Autodesk Fusion 360 part; units mm, degrees
(part 4 of 8)
  line L739 (-254.744, -72.9326) -> (-255.545, -72.9326)
  line L740 (-255.545, -72.9326) -> (-255.545, -69.8334)
  line L741 (-255.545, -69.8334) -> (-254.744, -69.8334)
  line L742 (-254.744, -69.8334) -> (-254.744, -64.0334)
  line L743 (-254.744, -64.0334) -> (-255.545, -64.0334)
  line L744 (-255.545, -64.0334) -> (-255.545, -60.9328)
  line L745 (-255.545, -60.9328) -> (-254.744, -60.9328)
  line L746 (-254.744, -60.9328) -> (-254.744, -59.9338)
  line L747 (-254.744, -59.9338) -> (-240.745, -59.9338)
  line L748 (-240.745, -59.9338) -> (-240.745, -60.9328)
  line L749 (-240.745, -60.9328) -> (-239.944, -60.9328)
  line L750 (-239.944, -60.9328) -> (-239.944, -64.0334)
  line L751 (-239.944, -64.0334) -> (-240.745, -64.0334)
  line L752 (-240.745, -64.0334) -> (-240.745, -69.8334)
  line L753 (-240.745, -69.8334) -> (-239.944, -69.8334)
  line L754 (-239.944, -69.8334) -> (-239.944, -72.9326)
  line L755 (-239.944, -72.9326) -> (-240.745, -72.9326)
  line L756 (-252.65, -35.833) -> (-266.65, -35.833)
  line L757 (-266.65, -35.833) -> (-266.65, -31.1326)
  line L758 (-266.65, -31.1326) -> (-268.176, -31.1326)
  line L759 (-268.176, -31.1326) -> (-268.176, -34.3628)
  line L760 (-268.176, -34.3628) -> (-274.925, -34.3628)
  line L761 (-274.925, -34.3628) -> (-274.925, -31.1326)
  line L762 (-274.925, -31.1326) -> (-275.751, -31.1326)
  line L763 (-275.751, -31.1326) -> (-275.751, -28.3338)
  line L764 (-275.751, -28.3338) -> (-274.925, -28.3338)
  line L765 (-274.925, -28.3338) -> (-274.925, -22.0638)
  line L766 (-274.925, -22.0638) -> (-273.2, -22.0638)
  line L767 (-273.2, -22.0638) -> (-273.2, -20.8635)
  line L768 (-273.2, -20.8635) -> (-269.9, -20.8635)
  line L769 (-269.9, -20.8635) -> (-269.9, -22.0638)
  line L770 (-269.9, -22.0638) -> (-268.176, -22.0638)
  line L771 (-268.176, -22.0638) -> (-268.176, -26.5327)
  line L772 (-268.176, -26.5327) -> (-266.65, -26.5327)
  line L773 (-266.65, -26.5327) -> (-266.65, -21.8336)
  line L774 (-266.65, -21.8336) -> (-252.65, -21.8336)
  line L775 (-252.65, -21.8336) -> (-252.65, -26.5327)
  line L776 (-252.65, -26.5327) -> (-251.126, -26.5327)
  line L777 (-251.126, -26.5327) -> (-251.126, -22.0638)
  line L778 (-251.126, -22.0638) -> (-249.4, -22.0638)
  line L779 (-249.4, -22.0638) -> (-249.4, -20.8635)
  line L780 (-249.4, -20.8635) -> (-246.101, -20.8635)
  line L781 (-246.101, -20.8635) -> (-246.101, -22.0638)
  line L782 (-246.101, -22.0638) -> (-244.376, -22.0638)
  line L783 (-244.376, -22.0638) -> (-244.376, -28.3338)
  line L784 (-244.376, -28.3338) -> (-243.55, -28.3338)
  line L785 (-243.55, -28.3338) -> (-243.55, -31.1326)
  line L786 (-243.55, -31.1326) -> (-244.376, -31.1326)
  line L787 (-244.376, -31.1326) -> (-244.376, -34.3628)
  line L788 (-244.376, -34.3628) -> (-251.126, -34.3628)
  line L789 (-251.126, -34.3628) -> (-251.126, -31.1326)
  line L790 (-251.126, -31.1326) -> (-252.65, -31.1326)
  line L791 (-252.65, -31.1326) -> (-252.65, -35.833)
  line L792 (-174.07, -91.9826) -> (-174.07, -92.9831)
  line L793 (-174.07, -92.9831) -> (-188.069, -92.9831)
  line L794 (-188.069, -92.9831) -> (-188.069, -91.9826)
  line L795 (-188.069, -91.9826) -> (-188.87, -91.9826)
  line L796 (-188.87, -91.9826) -> (-188.87, -88.8834)
  line L797 (-188.87, -88.8834) -> (-188.069, -88.8834)
  line L798 (-188.069, -88.8834) -> (-188.069, -83.0834)
  line L799 (-188.069, -83.0834) -> (-188.87, -83.0834)
  line L800 (-188.87, -83.0834) -> (-188.87, -79.9828)
  line L801 (-188.87, -79.9828) -> (-188.069, -79.9828)
  line L802 (-188.069, -79.9828) -> (-188.069, -78.9838)
  line L803 (-188.069, -78.9838) -> (-174.07, -78.9838)
  line L804 (-174.07, -78.9838) -> (-174.07, -79.9828)
  line L805 (-174.07, -79.9828) -> (-173.269, -79.9828)
  line L806 (-173.269, -79.9828) -> (-173.269, -83.0834)
  line L807 (-173.269, -83.0834) -> (-174.07, -83.0834)
  line L808 (-174.07, -83.0834) -> (-174.07, -88.8834)
  line L809 (-174.07, -88.8834) -> (-173.269, -88.8834)
  line L810 (-173.269, -88.8834) -> (-173.269, -91.9826)
  line L811 (-173.269, -91.9826) -> (-174.07, -91.9826)
  line L812 (-188.357, -53.8826) -> (-188.357, -54.8831)
  line L813 (-188.357, -54.8831) -> (-202.357, -54.8831)
  line L814 (-202.357, -54.8831) -> (-202.357, -53.8826)
  line L815 (-202.357, -53.8826) -> (-203.156, -53.8826)
  line L816 (-203.156, -53.8826) -> (-203.156, -50.7834)
  line L817 (-203.156, -50.7834) -> (-202.357, -50.7834)
  line L818 (-202.357, -50.7834) -> (-202.357, -44.9834)
  line L819 (-202.357, -44.9834) -> (-203.156, -44.9834)
  line L820 (-203.156, -44.9834) -> (-203.156, -41.8828)
  line L821 (-203.156, -41.8828) -> (-202.357, -41.8828)
  line L822 (-202.357, -41.8828) -> (-202.357, -40.8838)
  line L823 (-202.357, -40.8838) -> (-188.357, -40.8838)
  line L824 (-188.357, -40.8838) -> (-188.357, -41.8828)
  line L825 (-188.357, -41.8828) -> (-187.556, -41.8828)
  line L826 (-187.556, -41.8828) -> (-187.556, -44.9834)
  line L827 (-187.556, -44.9834) -> (-188.357, -44.9834)
  line L828 (-188.357, -44.9834) -> (-188.357, -50.7834)
  line L829 (-188.357, -50.7834) -> (-187.556, -50.7834)
  line L830 (-187.556, -50.7834) -> (-187.556, -53.8826)
  line L831 (-187.556, -53.8826) -> (-188.357, -53.8826)
  line L832 (-195.501, -15.7827) -> (-195.501, -16.7831)
  line L833 (-195.501, -16.7831) -> (-209.5, -16.7831)
  line L834 (-209.5, -16.7831) -> (-209.5, -15.7827)
  line L835 (-209.5, -15.7827) -> (-210.301, -15.7827)
  line L836 (-210.301, -15.7827) -> (-210.301, -12.6848)
  line L837 (-210.301, -12.6848) -> (-209.5, -12.6848)
  line L838 (-209.5, -12.6848) -> (-209.5, -6.8833)
  line L839 (-209.5, -6.8833) -> (-210.301, -6.8833)
  line L840 (-210.301, -6.8833) -> (-210.301, -3.7827)
  line L841 (-210.301, -3.7827) -> (-209.5, -3.7827)
  line L842 (-209.5, -3.7827) -> (-209.5, -2.7836)
  line L843 (-209.5, -2.7836) -> (-195.501, -2.7836)
  line L844 (-195.501, -2.7836) -> (-195.501, -3.7827)
  line L845 (-195.501, -3.7827) -> (-194.7, -3.7827)
  line L846 (-194.7, -3.7827) -> (-194.7, -6.8833)
  line L847 (-194.7, -6.8833) -> (-195.501, -6.8833)
  line L848 (-195.501, -6.8833) -> (-195.501, -12.6848)
  line L849 (-195.501, -12.6848) -> (-194.7, -12.6848)
  line L850 (-194.7, -12.6848) -> (-194.7, -15.7827)
  line L851 (-194.7, -15.7827) -> (-195.501, -15.7827)
  line L852 (-155.02, -91.9826) -> (-155.02, -92.9831)
  line L853 (-155.02, -92.9831) -> (-169.019, -92.9831)
  line L854 (-169.019, -92.9831) -> (-169.019, -91.9826)
  line L855 (-169.019, -91.9826) -> (-169.82, -91.9826)
  line L856 (-169.82, -91.9826) -> (-169.82, -88.8834)
  line L857 (-169.82, -88.8834) -> (-169.019, -88.8834)
  line L858 (-169.019, -88.8834) -> (-169.019, -83.0834)
  line L859 (-169.019, -83.0834) -> (-169.82, -83.0834)
  line L860 (-169.82, -83.0834) -> (-169.82, -79.9828)
  line L861 (-169.82, -79.9828) -> (-169.019, -79.9828)
  line L862 (-169.019, -79.9828) -> (-169.019, -78.9838)
  line L863 (-169.019, -78.9838) -> (-155.02, -78.9838)
  line L864 (-155.02, -78.9838) -> (-155.02, -79.9828)
  line L865 (-155.02, -79.9828) -> (-154.219, -79.9828)
  line L866 (-154.219, -79.9828) -> (-154.219, -83.0834)
  line L867 (-154.219, -83.0834) -> (-155.02, -83.0834)
  line L868 (-155.02, -83.0834) -> (-155.02, -88.8834)
  line L869 (-155.02, -88.8834) -> (-154.219, -88.8834)
  line L870 (-154.219, -88.8834) -> (-154.219, -91.9826)
  line L871 (-154.219, -91.9826) -> (-155.02, -91.9826)
  line L872 (-159.782, -34.8327) -> (-159.782, -35.833)
  line L873 (-159.782, -35.833) -> (-173.782, -35.833)
  line L874 (-173.782, -35.833) -> (-173.782, -34.8327)
  line L875 (-173.782, -34.8327) -> (-174.581, -34.8327)
  line L876 (-174.581, -34.8327) -> (-174.581, -31.7348)
  line L877 (-174.581, -31.7348) -> (-173.782, -31.7348)
  line L878 (-173.782, -31.7348) -> (-173.782, -25.9333)
  line L879 (-173.782, -25.9333) -> (-174.581, -25.9333)
  line L880 (-174.581, -25.9333) -> (-174.581, -22.8327)
  line L881 (-174.581, -22.8327) -> (-173.782, -22.8327)
  line L882 (-173.782, -22.8327) -> (-173.782, -21.8336)
  line L883 (-173.782, -21.8336) -> (-159.782, -21.8336)
  line L884 (-159.782, -21.8336) -> (-159.782, -22.8327)
  line L885 (-159.782, -22.8327) -> (-158.981, -22.8327)
  line L886 (-158.981, -22.8327) -> (-158.981, -25.9333)
  line L887 (-158.981, -25.9333) -> (-159.782, -25.9333)
  line L888 (-159.782, -25.9333) -> (-159.782, -31.7348)
  line L889 (-159.782, -31.7348) -> (-158.981, -31.7348)
  line L890 (-158.981, -31.7348) -> (-158.981, -34.8327)
  line L891 (-158.981, -34.8327) -> (-159.782, -34.8327)
  line L892 (-116.918, -91.9826) -> (-116.918, -92.9831)
  line L893 (-116.918, -92.9831) -> (-130.919, -92.9831)
  line L894 (-130.919, -92.9831) -> (-130.919, -91.9826)
  line L895 (-130.919, -91.9826) -> (-131.72, -91.9826)
  line L896 (-131.72, -91.9826) -> (-131.72, -88.8834)
  line L897 (-131.72, -88.8834) -> (-130.919, -88.8834)
  line L898 (-130.919, -88.8834) -> (-130.919, -83.0834)
  line L899 (-130.919, -83.0834) -> (-131.72, -83.0834)
  line L900 (-131.72, -83.0834) -> (-131.72, -79.9828)
  line L901 (-131.72, -79.9828) -> (-130.919, -79.9828)
  line L902 (-130.919, -79.9828) -> (-130.919, -78.9838)
  line L903 (-130.919, -78.9838) -> (-116.918, -78.9838)
  line L904 (-116.918, -78.9838) -> (-116.918, -79.9828)
  line L905 (-116.918, -79.9828) -> (-116.119, -79.9828)
  line L906 (-116.119, -79.9828) -> (-116.119, -83.0834)
  line L907 (-116.119, -83.0834) -> (-116.918, -83.0834)
  line L908 (-116.918, -83.0834) -> (-116.918, -88.8834)
  line L909 (-116.918, -88.8834) -> (-116.119, -88.8834)
  line L910 (-116.119, -88.8834) -> (-116.119, -91.9826)
  line L911 (-116.119, -91.9826) -> (-116.918, -91.9826)
  line L912 (-121.682, -34.8327) -> (-121.682, -35.833)
  line L913 (-121.682, -35.833) -> (-135.682, -35.833)
  line L914 (-135.682, -35.833) -> (-135.682, -34.8327)
  line L915 (-135.682, -34.8327) -> (-136.481, -34.8327)
  line L916 (-136.481, -34.8327) -> (-136.481, -31.7348)
  line L917 (-136.481, -31.7348) -> (-135.682, -31.7348)
  line L918 (-135.682, -31.7348) -> (-135.682, -25.9333)
  line L919 (-135.682, -25.9333) -> (-136.481, -25.9333)
  line L920 (-136.481, -25.9333) -> (-136.481, -22.8327)
  line L921 (-136.481, -22.8327) -> (-135.682, -22.8327)
  line L922 (-135.682, -22.8327) -> (-135.682, -21.8336)
  line L923 (-135.682, -21.8336) -> (-121.682, -21.8336)
  line L924 (-121.682, -21.8336) -> (-121.682, -22.8327)
  line L925 (-121.682, -22.8327) -> (-120.881, -22.8327)
  line L926 (-120.881, -22.8327) -> (-120.881, -25.9333)
  line L927 (-120.881, -25.9333) -> (-121.682, -25.9333)
  line L928 (-121.682, -25.9333) -> (-121.682, -31.7348)
  line L929 (-121.682, -31.7348) -> (-120.881, -31.7348)
  line L930 (-120.881, -31.7348) -> (-120.881, -34.8327)
  line L931 (-120.881, -34.8327) -> (-121.682, -34.8327)
  line L932 (-78.8197, -91.9826) -> (-78.8197, -92.9831)
  line L933 (-78.8197, -92.9831) -> (-92.819, -92.9831)
  line L934 (-92.819, -92.9831) -> (-92.819, -91.9826)
  line L935 (-92.819, -91.9826) -> (-93.6184, -91.9826)
  line L936 (-93.6184, -91.9826) -> (-93.6184, -88.8834)
  line L937 (-93.6184, -88.8834) -> (-92.819, -88.8834)
  line L938 (-92.819, -88.8834) -> (-92.819, -83.0834)
  line L939 (-92.819, -83.0834) -> (-93.6184, -83.0834)
  line L940 (-93.6184, -83.0834) -> (-93.6184, -79.9828)
  line L941 (-93.6184, -79.9828) -> (-92.819, -79.9828)
  line L942 (-92.819, -79.9828) -> (-92.819, -78.9838)
  line L943 (-92.819, -78.9838) -> (-78.8197, -78.9838)
  line L944 (-78.8197, -78.9838) -> (-78.8197, -79.9828)
  line L945 (-78.8197, -79.9828) -> (-78.0189, -79.9828)
  line L946 (-78.0189, -79.9828) -> (-78.0189, -83.0834)
  line L947 (-78.0189, -83.0834) -> (-78.8197, -83.0834)
  line L948 (-78.8197, -83.0834) -> (-78.8197, -88.8834)
  line L949 (-78.8197, -88.8834) -> (-78.0189, -88.8834)
  line L950 (-78.0189, -88.8834) -> (-78.0189, -91.9826)
  line L951 (-78.0189, -91.9826) -> (-78.8197, -91.9826)
  line L952 (-83.5822, -34.8327) -> (-83.5822, -35.833)
  line L953 (-83.5822, -35.833) -> (-97.5815, -35.833)
  line L954 (-97.5815, -35.833) -> (-97.5815, -34.8327)
  line L955 (-97.5815, -34.8327) -> (-98.3809, -34.8327)
  line L956 (-98.3809, -34.8327) -> (-98.3809, -31.7348)
  line L957 (-98.3809, -31.7348) -> (-97.5815, -31.7348)
  line L958 (-97.5815, -31.7348) -> (-97.5815, -25.9333)
  line L959 (-97.5815, -25.9333) -> (-98.3809, -25.9333)
  line L960 (-98.3809, -25.9333) -> (-98.3809, -22.8327)
  line L961 (-98.3809, -22.8327) -> (-97.5815, -22.8327)
  line L962 (-97.5815, -22.8327) -> (-97.5815, -21.8336)
  line L963 (-97.5815, -21.8336) -> (-83.5822, -21.8336)
  line L964 (-83.5822, -21.8336) -> (-83.5822, -22.8327)
  line L965 (-83.5822, -22.8327) -> (-82.7814, -22.8327)
  line L966 (-82.7814, -22.8327) -> (-82.7814, -25.9333)
  line L967 (-82.7814, -25.9333) -> (-83.5822, -25.9333)
  line L968 (-83.5822, -25.9333) -> (-83.5822, -31.7348)
  line L969 (-83.5822, -31.7348) -> (-82.7814, -31.7348)
  line L970 (-82.7814, -31.7348) -> (-82.7814, -34.8327)
  line L971 (-82.7814, -34.8327) -> (-83.5822, -34.8327)
  line L972 (-50.2447, -72.9326) -> (-50.2447, -73.9331)
  line L973 (-50.2447, -73.9331) -> (-64.244, -73.9331)
  line L974 (-64.244, -73.9331) -> (-64.244, -72.9326)
  line L975 (-64.244, -72.9326) -> (-65.0448, -72.9326)
  line L976 (-65.0448, -72.9326) -> (-65.0448, -69.8334)
  line L977 (-65.0448, -69.8334) -> (-64.244, -69.8334)
  line L978 (-64.244, -69.8334) -> (-64.244, -64.0334)
  line L979 (-64.244, -64.0334) -> (-65.0448, -64.0334)
  line L980 (-65.0448, -64.0334) -> (-65.0448, -60.9328)
  line L981 (-65.0448, -60.9328) -> (-64.244, -60.9328)
  line L982 (-64.244, -60.9328) -> (-64.244, -59.9338)
  line L983 (-64.244, -59.9338) -> (-50.2447, -59.9338)
  line L984 (-50.2447, -59.9338) -> (-50.2447, -60.9328)
  line L985 (-50.2447, -60.9328) -> (-49.4439, -60.9328)
  line L986 (-49.4439, -60.9328) -> (-49.4439, -64.0334)
  line L987 (-49.4439, -64.0334) -> (-50.2447, -64.0334)
  line L988 (-50.2447, -64.0334) -> (-50.2447, -69.8334)
  line L989 (-50.2447, -69.8334) -> (-49.4439, -69.8334)
  line L990 (-49.4439, -69.8334) -> (-49.4439, -72.9326)
  line L991 (-49.4439, -72.9326) -> (-50.2447, -72.9326)
  line L992 (-45.4822, -34.8327) -> (-45.4822, -35.833)
  line L993 (-45.4822, -35.833) -> (-59.4815, -35.833)
  line L994 (-59.4815, -35.833) -> (-59.4815, -34.8327)
  line L995 (-59.4815, -34.8327) -> (-60.2809, -34.8327)
  line L996 (-60.2809, -34.8327) -> (-60.2809, -31.7348)
  line L997 (-60.2809, -31.7348) -> (-59.4815, -31.7348)
  line L998 (-59.4815, -31.7348) -> (-59.4815, -25.9333)
  line L999 (-59.4815, -25.9333) -> (-60.2809, -25.9333)
  line L1000 (-60.2809, -25.9333) -> (-60.2809, -22.8327)
  line L1001 (-60.2809, -22.8327) -> (-59.4815, -22.8327)
  line L1002 (-59.4815, -22.8327) -> (-59.4815, -21.8336)
  line L1003 (-59.4815, -21.8336) -> (-45.4822, -21.8336)
  line L1004 (-45.4822, -21.8336) -> (-45.4822, -22.8327)
  line L1005 (-45.4822, -22.8327) -> (-44.6814, -22.8327)
  line L1006 (-44.6814, -22.8327) -> (-44.6814, -25.9333)
  line L1007 (-44.6814, -25.9333) -> (-45.4822, -25.9333)
  line L1008 (-45.4822, -25.9333) -> (-45.4822, -31.7348)
  line L1009 (-45.4822, -31.7348) -> (-44.6814, -31.7348)
  line L1010 (-44.6814, -31.7348) -> (-44.6814, -34.8327)
  line L1011 (-44.6814, -34.8327) -> (-45.4822, -34.8327)
  line L1012 (-14.5259, -35.833) -> (-28.5254, -35.833)
  line L1013 (-28.5254, -35.833) -> (-28.5254, -31.1326)
  line L1014 (-28.5254, -31.1326) -> (-30.0509, -31.1326)
  line L1015 (-30.0509, -31.1326) -> (-30.0509, -34.3628)
  line L1016 (-30.0509, -34.3628) -> (-36.8004, -34.3628)
  line L1017 (-36.8004, -34.3628) -> (-36.8004, -31.1326)
  line L1018 (-36.8004, -31.1326) -> (-37.6259, -31.1326)
  line L1019 (-37.6259, -31.1326) -> (-37.6259, -28.3338)
  line L1020 (-37.6259, -28.3338) -> (-36.8004, -28.3338)
  line L1021 (-36.8004, -28.3338) -> (-36.8004, -22.0638)
  line L1022 (-36.8004, -22.0638) -> (-35.0752, -22.0638)
  line L1023 (-35.0752, -22.0638) -> (-35.0752, -20.8635)
  line L1024 (-35.0752, -20.8635) -> (-31.7748, -20.8635)
  line L1025 (-31.7748, -20.8635) -> (-31.7748, -22.0638)
  line L1026 (-31.7748, -22.0638) -> (-30.0509, -22.0638)
  line L1027 (-30.0509, -22.0638) -> (-30.0509, -26.5327)
  line L1028 (-30.0509, -26.5327) -> (-28.5254, -26.5327)
  line L1029 (-28.5254, -26.5327) -> (-28.5254, -21.8336)
  line L1030 (-28.5254, -21.8336) -> (-14.5259, -21.8336)
  line L1031 (-14.5259, -21.8336) -> (-14.5259, -26.5327)
  line L1032 (-14.5259, -26.5327) -> (-13.0004, -26.5327)
  line L1033 (-13.0004, -26.5327) -> (-13.0004, -22.0638)
  line L1034 (-13.0004, -22.0638) -> (-11.2751, -22.0638)
  line L1035 (-11.2751, -22.0638) -> (-11.2751, -20.8635)
  line L1036 (-11.2751, -20.8635) -> (-7.9761, -20.8635)
  line L1037 (-7.9761, -20.8635) -> (-7.9761, -22.0638)
  line L1038 (-7.9761, -22.0638) -> (-6.2508, -22.0638)
  line L1039 (-6.2508, -22.0638) -> (-6.2508, -28.3338)
  line L1040 (-6.2508, -28.3338) -> (-5.4253, -28.3338)
  line L1041 (-5.4253, -28.3338) -> (-5.4253, -31.1326)
  line L1042 (-5.4253, -31.1326) -> (-6.2508, -31.1326)
  line L1043 (-6.2508, -31.1326) -> (-6.2508, -34.3628)
  line L1044 (-6.2508, -34.3628) -> (-13.0004, -34.3628)
  line L1045 (-13.0004, -34.3628) -> (-13.0004, -31.1326)
  line L1046 (-13.0004, -31.1326) -> (-14.5259, -31.1326)
  line L1047 (-14.5259, -31.1326) -> (-14.5259, -35.833)
  line L1048 (-7.3822, -72.9326) -> (-7.3822, -73.9331)
  line L1049 (-7.3822, -73.9331) -> (-21.3817, -73.9331)
  line L1050 (-21.3817, -73.9331) -> (-21.3817, -72.9326)
  line L1051 (-21.3817, -72.9326) -> (-22.1809, -72.9326)
  line L1052 (-22.1809, -72.9326) -> (-22.1809, -69.8334)
  line L1053 (-22.1809, -69.8334) -> (-21.3817, -69.8334)
  line L1054 (-21.3817, -69.8334) -> (-21.3817, -64.0334)
  line L1055 (-21.3817, -64.0334) -> (-22.1809, -64.0334)
  line L1056 (-22.1809, -64.0334) -> (-22.1809, -60.9328)
  line L1057 (-22.1809, -60.9328) -> (-21.3817, -60.9328)
  line L1058 (-21.3817, -60.9328) -> (-21.3817, -59.9338)
  line L1059 (-21.3817, -59.9338) -> (-7.3822, -59.9338)
  line L1060 (-7.3822, -59.9338) -> (-7.3822, -60.9328)
  line L1061 (-7.3822, -60.9328) -> (-6.5815, -60.9328)
  line L1062 (-6.5815, -60.9328) -> (-6.5815, -64.0334)
  line L1063 (-6.5815, -64.0334) -> (-7.3822, -64.0334)
  line L1064 (-7.3822, -64.0334) -> (-7.3822, -69.8334)
  line L1065 (-7.3822, -69.8334) -> (-6.5815, -69.8334)
  line L1066 (-6.5815, -69.8334) -> (-6.5815, -72.9326)
  line L1067 (-6.5815, -72.9326) -> (-7.3822, -72.9326)
  line L1068 (-9.762, -53.8826) -> (-9.762, -54.8831)
  line L1069 (-9.762, -54.8831) -> (-23.7629, -54.8831)
  line L1070 (-23.7629, -54.8831) -> (-23.7629, -53.8826)
  line L1071 (-23.7629, -53.8826) -> (-24.5622, -53.8826)
  line L1072 (-24.5622, -53.8826) -> (-24.5622, -50.7834)
  line L1073 (-24.5622, -50.7834) -> (-23.7629, -50.7834)
  line L1074 (-23.7629, -50.7834) -> (-23.7629, -44.9834)
  line L1075 (-23.7629, -44.9834) -> (-24.5622, -44.9834)
  line L1076 (-24.5622, -44.9834) -> (-24.5622, -41.8828)
  line L1077 (-24.5622, -41.8828) -> (-23.7629, -41.8828)
  line L1078 (-23.7629, -41.8828) -> (-23.7629, -40.8838)
  line L1079 (-23.7629, -40.8838) -> (-9.762, -40.8838)
  line L1080 (-9.762, -40.8838) -> (-9.762, -41.8828)
  line L1081 (-9.762, -41.8828) -> (-8.9628, -41.8828)
  line L1082 (-8.9628, -41.8828) -> (-8.9628, -44.9834)
  line L1083 (-8.9628, -44.9834) -> (-9.762, -44.9834)
  line L1084 (-9.762, -44.9834) -> (-9.762, -50.7834)
  line L1085 (-9.762, -50.7834) -> (-8.9628, -50.7834)
  line L1086 (-8.9628, -50.7834) -> (-8.9628, -53.8826)
  line L1087 (-8.9628, -53.8826) -> (-9.762, -53.8826)
  line L1088 (-52.626, -15.7827) -> (-52.626, -16.7831)
  line L1089 (-52.626, -16.7831) -> (-66.6253, -16.7831)
  line L1090 (-66.6253, -16.7831) -> (-66.6253, -15.7827)
  line L1091 (-66.6253, -15.7827) -> (-67.4261, -15.7827)
  line L1092 (-67.4261, -15.7827) -> (-67.4261, -12.6848)
  line L1093 (-67.4261, -12.6848) -> (-66.6253, -12.6848)
  line L1094 (-66.6253, -12.6848) -> (-66.6253, -6.8833)
  line L1095 (-66.6253, -6.8833) -> (-67.4261, -6.8833)
  line L1096 (-67.4261, -6.8833) -> (-67.4261, -3.7827)
  line L1097 (-67.4261, -3.7827) -> (-66.6253, -3.7827)
  line L1098 (-66.6253, -3.7827) -> (-66.6253, -2.7836)
  line L1099 (-66.6253, -2.7836) -> (-52.626, -2.7836)
  line L1100 (-52.626, -2.7836) -> (-52.626, -3.7827)
  line L1101 (-52.626, -3.7827) -> (-51.8252, -3.7827)
  line L1102 (-51.8252, -3.7827) -> (-51.8252, -6.8833)
  line L1103 (-51.8252, -6.8833) -> (-52.626, -6.8833)
  line L1104 (-52.626, -6.8833) -> (-52.626, -12.6848)
  line L1105 (-52.626, -12.6848) -> (-51.8252, -12.6848)
  line L1106 (-51.8252, -12.6848) -> (-51.8252, -15.7827)
  line L1107 (-51.8252, -15.7827) -> (-52.626, -15.7827)
  line L1108 (-40.7197, -91.9826) -> (-40.7197, -92.9831)
  line L1109 (-40.7197, -92.9831) -> (-54.719, -92.9831)
  line L1110 (-54.719, -92.9831) -> (-54.719, -91.9826)
  line L1111 (-54.719, -91.9826) -> (-55.5198, -91.9826)
  line L1112 (-55.5198, -91.9826) -> (-55.5198, -88.8834)
  line L1113 (-55.5198, -88.8834) -> (-54.719, -88.8834)
  line L1114 (-54.719, -88.8834) -> (-54.719, -83.0834)
  line L1115 (-54.719, -83.0834) -> (-55.5198, -83.0834)
  line L1116 (-55.5198, -83.0834) -> (-55.5198, -79.9828)
  line L1117 (-55.5198, -79.9828) -> (-54.719, -79.9828)
  line L1118 (-54.719, -79.9828) -> (-54.719, -78.9838)
  line L1119 (-54.719, -78.9838) -> (-40.7197, -78.9838)
  line L1120 (-40.7197, -78.9838) -> (-40.7197, -79.9828)
  line L1121 (-40.7197, -79.9828) -> (-39.9189, -79.9828)
  line L1122 (-39.9189, -79.9828) -> (-39.9189, -83.0834)
  line L1123 (-39.9189, -83.0834) -> (-40.7197, -83.0834)
  line L1124 (-40.7197, -83.0834) -> (-40.7197, -88.8834)
  line L1125 (-40.7197, -88.8834) -> (-39.9189, -88.8834)
  line L1126 (-39.9189, -88.8834) -> (-39.9189, -91.9826)
  line L1127 (-39.9189, -91.9826) -> (-40.7197, -91.9826)
  line L1128 (-124.062, -15.7827) -> (-124.062, -16.7831)
  line L1129 (-124.062, -16.7831) -> (-138.063, -16.7831)
  line L1130 (-138.063, -16.7831) -> (-138.063, -15.7827)
  line L1131 (-138.063, -15.7827) -> (-138.862, -15.7827)
  line L1132 (-138.862, -15.7827) -> (-138.862, -12.6848)
  line L1133 (-138.862, -12.6848) -> (-138.063, -12.6848)
  line L1134 (-138.063, -12.6848) -> (-138.063, -12.0826)
  line L1135 (-138.063, -12.0826) -> (-177.687, -12.0826)
  line L1136 (-177.687, -12.0826) -> (-177.687, -15.3128)
  line L1137 (-177.687, -15.3128) -> (-184.438, -15.3128)
  line L1138 (-184.438, -15.3128) -> (-184.438, -12.0826)
  line L1139 (-184.438, -12.0826) -> (-185.262, -12.0826)
  line L1140 (-185.262, -12.0826) -> (-185.262, -9.2838)
  line L1141 (-185.262, -9.2838) -> (-184.438, -9.2838)
  line L1142 (-184.438, -9.2838) -> (-184.438, -3.0138)
  line L1143 (-184.438, -3.0138) -> (-182.713, -3.0138)
  line L1144 (-182.713, -3.0138) -> (-182.713, -1.8135)
  line L1145 (-182.713, -1.8135) -> (-179.412, -1.8135)
  line L1146 (-179.412, -1.8135) -> (-179.412, -3.0138)
  line L1147 (-179.412, -3.0138) -> (-177.687, -3.0138)
  line L1148 (-177.687, -3.0138) -> (-177.687, -7.4841)
  line L1149 (-177.687, -7.4841) -> (-138.063, -7.4841)
  line L1150 (-138.063, -7.4841) -> (-138.063, -6.8833)
  line L1151 (-138.063, -6.8833) -> (-138.862, -6.8833)
  line L1152 (-138.862, -6.8833) -> (-138.862, -3.7827)
  line L1153 (-138.862, -3.7827) -> (-138.063, -3.7827)
  line L1154 (-138.063, -3.7827) -> (-138.063, -2.7836)
  line L1155 (-138.063, -2.7836) -> (-124.062, -2.7836)
  line L1156 (-124.062, -2.7836) -> (-124.062, -3.7827)
  line L1157 (-124.062, -3.7827) -> (-123.263, -3.7827)
  line L1158 (-123.263, -3.7827) -> (-123.263, -6.8833)
  line L1159 (-123.263, -6.8833) -> (-124.062, -6.8833)
  line L1160 (-124.062, -6.8833) -> (-124.062, -7.4841)
  line L1161 (-124.062, -7.4841) -> (-84.4381, -7.4841)
  line L1162 (-84.4381, -7.4841) -> (-84.4381, -3.0138)
  line L1163 (-84.4381, -3.0138) -> (-82.7126, -3.0138)
  line L1164 (-82.7126, -3.0138) -> (-82.7126, -1.8135)
  line L1165 (-82.7126, -1.8135) -> (-79.412, -1.8135)
  line L1166 (-79.412, -1.8135) -> (-79.412, -3.0138)
  line L1167 (-79.412, -3.0138) -> (-77.687, -3.0138)
  line L1168 (-77.687, -3.0138) -> (-77.687, -9.2838)
  line L1169 (-77.687, -9.2838) -> (-76.8629, -9.2838)
  line L1170 (-76.8629, -9.2838) -> (-76.8629, -12.0826)
  line L1171 (-76.8629, -12.0826) -> (-77.687, -12.0826)
  line L1172 (-77.687, -12.0826) -> (-77.687, -15.3128)
  line L1173 (-77.687, -15.3128) -> (-84.4381, -15.3128)
  line L1174 (-84.4381, -15.3128) -> (-84.4381, -12.0826)
  line L1175 (-84.4381, -12.0826) -> (-124.062, -12.0826)
  line L1176 (-124.062, -12.0826) -> (-124.062, -12.6848)
  line L1177 (-124.062, -12.6848) -> (-123.263, -12.6848)
  line L1178 (-123.263, -12.6848) -> (-123.263, -15.7827)
  line L1179 (-123.263, -15.7827) -> (-124.062, -15.7827)
  line L1180 (-59.7697, -91.9826) -> (-59.7697, -92.9831)
  line L1181 (-59.7697, -92.9831) -> (-73.769, -92.9831)
  line L1182 (-73.769, -92.9831) -> (-73.769, -91.9826)
  line L1183 (-73.769, -91.9826) -> (-74.5698, -91.9826)
  line L1184 (-74.5698, -91.9826) -> (-74.5698, -88.8834)
  line L1185 (-74.5698, -88.8834) -> (-73.769, -88.8834)
  line L1186 (-73.769, -88.8834) -> (-73.769, -83.0834)
  line L1187 (-73.769, -83.0834) -> (-74.5698, -83.0834)
  line L1188 (-74.5698, -83.0834) -> (-74.5698, -79.9828)
  line L1189 (-74.5698, -79.9828) -> (-73.769, -79.9828)
  line L1190 (-73.769, -79.9828) -> (-73.769, -78.9838)
  line L1191 (-73.769, -78.9838) -> (-59.7697, -78.9838)
  line L1192 (-59.7697, -78.9838) -> (-59.7697, -79.9828)
  line L1193 (-59.7697, -79.9828) -> (-58.9689, -79.9828)
  line L1194 (-58.9689, -79.9828) -> (-58.9689, -83.0834)
  line L1195 (-58.9689, -83.0834) -> (-59.7697, -83.0834)
  line L1196 (-59.7697, -83.0834) -> (-59.7697, -88.8834)
  line L1197 (-59.7697, -88.8834) -> (-58.9689, -88.8834)
  line L1198 (-58.9689, -88.8834) -> (-58.9689, -91.9826)
  line L1199 (-58.9689, -91.9826) -> (-59.7697, -91.9826)
  line L1200 (-102.632, -34.8327) -> (-102.632, -35.833)
  line L1201 (-102.632, -35.833) -> (-116.632, -35.833)
  line L1202 (-116.632, -35.833) -> (-116.632, -34.8327)
  line L1203 (-116.632, -34.8327) -> (-117.431, -34.8327)
  line L1204 (-117.431, -34.8327) -> (-117.431, -31.7348)
  line L1205 (-117.431, -31.7348) -> (-116.632, -31.7348)
  line L1206 (-116.632, -31.7348) -> (-116.632, -25.9333)
  line L1207 (-116.632, -25.9333) -> (-117.431, -25.9333)
  line L1208 (-117.431, -25.9333) -> (-117.431, -22.8327)
  line L1209 (-117.431, -22.8327) -> (-116.632, -22.8327)
  line L1210 (-116.632, -22.8327) -> (-116.632, -21.8336)
  line L1211 (-116.632, -21.8336) -> (-102.632, -21.8336)
  line L1212 (-102.632, -21.8336) -> (-102.632, -22.8327)
  line L1213 (-102.632, -22.8327) -> (-101.831, -22.8327)
  line L1214 (-101.831, -22.8327) -> (-101.831, -25.9333)
  line L1215 (-101.831, -25.9333) -> (-102.632, -25.9333)
  line L1216 (-102.632, -25.9333) -> (-102.632, -31.7348)
  line L1217 (-102.632, -31.7348) -> (-101.831, -31.7348)
  line L1218 (-101.831, -31.7348) -> (-101.831, -34.8327)
  line L1219 (-101.831, -34.8327) -> (-102.632, -34.8327)
  line L1220 (-97.8683, -91.9826) -> (-97.8683, -92.9831)
  line L1221 (-97.8683, -92.9831) -> (-111.869, -92.9831)
  line L1222 (-111.869, -92.9831) -> (-111.869, -91.9826)
  line L1223 (-111.869, -91.9826) -> (-112.668, -91.9826)
  line L1224 (-112.668, -91.9826) -> (-112.668, -88.8834)
  line L1225 (-112.668, -88.8834) -> (-111.869, -88.8834)
  line L1226 (-111.869, -88.8834) -> (-111.869, -83.0834)
  line L1227 (-111.869, -83.0834) -> (-112.668, -83.0834)
  line L1228 (-112.668, -83.0834) -> (-112.668, -79.9828)
  line L1229 (-112.668, -79.9828) -> (-111.869, -79.9828)
  line L1230 (-111.869, -79.9828) -> (-111.869, -78.9838)
  line L1231 (-111.869, -78.9838) -> (-97.8683, -78.9838)
  line L1232 (-97.8683, -78.9838) -> (-97.8683, -79.9828)
  line L1233 (-97.8683, -79.9828) -> (-97.0689, -79.9828)
  line L1234 (-97.0689, -79.9828) -> (-97.0689, -83.0834)
  line L1235 (-97.0689, -83.0834) -> (-97.8683, -83.0834)
  line L1236 (-97.8683, -83.0834) -> (-97.8683, -88.8834)
  line L1237 (-97.8683, -88.8834) -> (-97.0689, -88.8834)
  line L1238 (-97.0689, -88.8834) -> (-97.0689, -91.9826)
  line L1239 (-97.0689, -91.9826) -> (-97.8683, -91.9826)
  line L1240 (-140.732, -34.8327) -> (-140.732, -35.833)
  line L1241 (-140.732, -35.833) -> (-154.732, -35.833)
  line L1242 (-154.732, -35.833) -> (-154.732, -34.8327)
  line L1243 (-154.732, -34.8327) -> (-155.531, -34.8327)
  line L1244 (-155.531, -34.8327) -> (-155.531, -31.7348)
  line L1245 (-155.531, -31.7348) -> (-154.732, -31.7348)
  line L1246 (-154.732, -31.7348) -> (-154.732, -25.9333)
  line L1247 (-154.732, -25.9333) -> (-155.531, -25.9333)
  line L1248 (-155.531, -25.9333) -> (-155.531, -22.8327)
  line L1249 (-155.531, -22.8327) -> (-154.732, -22.8327)
  line L1250 (-154.732, -22.8327) -> (-154.732, -21.8336)
  line L1251 (-154.732, -21.8336) -> (-140.732, -21.8336)
  line L1252 (-140.732, -21.8336) -> (-140.732, -22.8327)
  line L1253 (-140.732, -22.8327) -> (-139.931, -22.8327)
  line L1254 (-139.931, -22.8327) -> (-139.931, -25.9333)
  line L1255 (-139.931, -25.9333) -> (-140.732, -25.9333)
  line L1256 (-140.732, -25.9333) -> (-140.732, -31.7348)
  line L1257 (-140.732, -31.7348) -> (-139.931, -31.7348)
  line L1258 (-139.931, -31.7348) -> (-139.931, -34.8327)
  line L1259 (-139.931, -34.8327) -> (-140.732, -34.8327)
  line L1260 (-135.97, -91.9826) -> (-135.97, -92.9831)
  line L1261 (-135.97, -92.9831) -> (-149.969, -92.9831)
  line L1262 (-149.969, -92.9831) -> (-149.969, -91.9826)
  line L1263 (-149.969, -91.9826) -> (-150.77, -91.9826)
  line L1264 (-150.77, -91.9826) -> (-150.77, -88.8834)
  line L1265 (-150.77, -88.8834) -> (-149.969, -88.8834)
  line L1266 (-149.969, -88.8834) -> (-149.969, -83.0834)
  line L1267 (-149.969, -83.0834) -> (-150.77, -83.0834)
  line L1268 (-150.77, -83.0834) -> (-150.77, -79.9828)
  line L1269 (-150.77, -79.9828) -> (-149.969, -79.9828)
  line L1270 (-149.969, -79.9828) -> (-149.969, -78.9838)
  line L1271 (-149.969, -78.9838) -> (-135.97, -78.9838)
  line L1272 (-135.97, -78.9838) -> (-135.97, -79.9828)
  line L1273 (-135.97, -79.9828) -> (-135.169, -79.9828)
  line L1274 (-135.169, -79.9828) -> (-135.169, -83.0834)
  line L1275 (-135.169, -83.0834) -> (-135.97, -83.0834)
  line L1276 (-135.97, -83.0834) -> (-135.97, -88.8834)
  line L1277 (-135.97, -88.8834) -> (-135.169, -88.8834)
  line L1278 (-135.169, -88.8834) -> (-135.169, -91.9826)
  line L1279 (-135.169, -91.9826) -> (-135.97, -91.9826)
  line L1280 (-178.832, -34.8327) -> (-178.832, -35.833)
  line L1281 (-178.832, -35.833) -> (-192.832, -35.833)
  line L1282 (-192.832, -35.833) -> (-192.832, -34.8327)
  line L1283 (-192.832, -34.8327) -> (-193.631, -34.8327)
  line L1284 (-193.631, -34.8327) -> (-193.631, -31.7348)
  line L1285 (-193.631, -31.7348) -> (-192.832, -31.7348)
  line L1286 (-192.832, -31.7348) -> (-192.832, -25.9333)
  line L1287 (-192.832, -25.9333) -> (-193.631, -25.9333)
  line L1288 (-193.631, -25.9333) -> (-193.631, -22.8327)
  line L1289 (-193.631, -22.8327) -> (-192.832, -22.8327)
  line L1290 (-192.832, -22.8327) -> (-192.832, -21.8336)
  line L1291 (-192.832, -21.8336) -> (-178.832, -21.8336)
  line L1292 (-178.832, -21.8336) -> (-178.832, -22.8327)
  line L1293 (-178.832, -22.8327) -> (-178.031, -22.8327)
  line L1294 (-178.031, -22.8327) -> (-178.031, -25.9333)
  line L1295 (-178.031, -25.9333) -> (-178.832, -25.9333)
  line L1296 (-178.832, -25.9333) -> (-178.832, -31.7348)
  line L1297 (-178.832, -31.7348) -> (-178.031, -31.7348)
  line L1298 (-178.031, -31.7348) -> (-178.031, -34.8327)
  line L1299 (-178.031, -34.8327) -> (-178.832, -34.8327)
  line L1300 (-197.882, -34.8327) -> (-197.882, -35.833)
  line L1301 (-197.882, -35.833) -> (-211.882, -35.833)
  line L1302 (-211.882, -35.833) -> (-211.882, -34.8327)
  line L1303 (-211.882, -34.8327) -> (-212.681, -34.8327)
  line L1304 (-212.681, -34.8327) -> (-212.681, -31.7348)
  line L1305 (-212.681, -31.7348) -> (-211.882, -31.7348)
  line L1306 (-211.882, -31.7348) -> (-211.882, -25.9333)
  line L1307 (-211.882, -25.9333) -> (-212.681, -25.9333)
  line L1308 (-212.681, -25.9333) -> (-212.681, -22.8327)
  line L1309 (-212.681, -22.8327) -> (-211.882, -22.8327)
  line L1310 (-211.882, -22.8327) -> (-211.882, -21.8336)
  line L1311 (-211.882, -21.8336) -> (-197.882, -21.8336)
  line L1312 (-197.882, -21.8336) -> (-197.882, -22.8327)
  line L1313 (-197.882, -22.8327) -> (-197.081, -22.8327)
  line L1314 (-197.081, -22.8327) -> (-197.081, -25.9333)
  line L1315 (-197.081, -25.9333) -> (-197.882, -25.9333)
  line L1316 (-197.882, -25.9333) -> (-197.882, -31.7348)
  line L1317 (-197.882, -31.7348) -> (-197.081, -31.7348)
  line L1318 (-197.081, -31.7348) -> (-197.081, -34.8327)
  line L1319 (-197.081, -34.8327) -> (-197.882, -34.8327)
  line L1320 (-183.595, -72.9326) -> (-183.595, -73.9331)
  line L1321 (-183.595, -73.9331) -> (-197.594, -73.9331)
  line L1322 (-197.594, -73.9331) -> (-197.594, -72.9326)
  line L1323 (-197.594, -72.9326) -> (-198.395, -72.9326)
  line L1324 (-198.395, -72.9326) -> (-198.395, -69.8334)
  line L1325 (-198.395, -69.8334) -> (-197.594, -69.8334)
  line L1326 (-197.594, -69.8334) -> (-197.594, -64.0334)
  line L1327 (-197.594, -64.0334) -> (-198.395, -64.0334)
  line L1328 (-198.395, -64.0334) -> (-198.395, -60.9328)
  line L1329 (-198.395, -60.9328) -> (-197.594, -60.9328)
  line L1330 (-197.594, -60.9328) -> (-197.594, -59.9338)
  line L1331 (-197.594, -59.9338) -> (-183.595, -59.9338)
  line L1332 (-183.595, -59.9338) -> (-183.595, -60.9328)
  line L1333 (-183.595, -60.9328) -> (-182.794, -60.9328)
  line L1334 (-182.794, -60.9328) -> (-182.794, -64.0334)
  line L1335 (-182.794, -64.0334) -> (-183.595, -64.0334)
  line L1336 (-183.595, -64.0334) -> (-183.595, -69.8334)
  line L1337 (-183.595, -69.8334) -> (-182.794, -69.8334)
  line L1338 (-182.794, -69.8334) -> (-182.794, -72.9326)
  line L1339 (-182.794, -72.9326) -> (-183.595, -72.9326)
  line L1340 (-226.457, -53.8826) -> (-226.457, -54.8831)
  line L1341 (-226.457, -54.8831) -> (-240.457, -54.8831)
  line L1342 (-240.457, -54.8831) -> (-240.457, -53.8826)
  line L1343 (-240.457, -53.8826) -> (-241.256, -53.8826)
  line L1344 (-241.256, -53.8826) -> (-241.256, -50.7834)
  line L1345 (-241.256, -50.7834) -> (-240.457, -50.7834)
  line L1346 (-240.457, -50.7834) -> (-240.457, -44.9834)
  line L1347 (-240.457, -44.9834) -> (-241.256, -44.9834)
  line L1348 (-241.256, -44.9834) -> (-241.256, -41.8828)
  line L1349 (-241.256, -41.8828) -> (-240.457, -41.8828)
  line L1350 (-240.457, -41.8828) -> (-240.457, -40.8838)
  line L1351 (-240.457, -40.8838) -> (-226.457, -40.8838)
  line L1352 (-226.457, -40.8838) -> (-226.457, -41.8828)
  line L1353 (-226.457, -41.8828) -> (-225.656, -41.8828)
  line L1354 (-225.656, -41.8828) -> (-225.656, -44.9834)
  line L1355 (-225.656, -44.9834) -> (-226.457, -44.9834)
  line L1356 (-226.457, -44.9834) -> (-226.457, -50.7834)
  line L1357 (-226.457, -50.7834) -> (-225.656, -50.7834)
  line L1358 (-225.656, -50.7834) -> (-225.656, -53.8826)
  line L1359 (-225.656, -53.8826) -> (-226.457, -53.8826)
  line L1360 (-221.695, -72.9326) -> (-221.695, -73.9331)
  line L1361 (-221.695, -73.9331) -> (-235.694, -73.9331)
  line L1362 (-235.694, -73.9331) -> (-235.694, -72.9326)
  line L1363 (-235.694, -72.9326) -> (-236.495, -72.9326)
  line L1364 (-236.495, -72.9326) -> (-236.495, -69.8334)
  line L1365 (-236.495, -69.8334) -> (-235.694, -69.8334)
  line L1366 (-235.694, -69.8334) -> (-235.694, -64.0334)
  line L1367 (-235.694, -64.0334) -> (-236.495, -64.0334)
  line L1368 (-236.495, -64.0334) -> (-236.495, -60.9328)
  line L1369 (-236.495, -60.9328) -> (-235.694, -60.9328)
  line L1370 (-235.694, -60.9328) -> (-235.694, -59.9338)
  line L1371 (-235.694, -59.9338) -> (-221.695, -59.9338)
  line L1372 (-221.695, -59.9338) -> (-221.695, -60.9328)
  line L1373 (-221.695, -60.9328) -> (-220.894, -60.9328)
  line L1374 (-220.894, -60.9328) -> (-220.894, -64.0334)
  line L1375 (-220.894, -64.0334) -> (-221.695, -64.0334)
  line L1376 (-221.695, -64.0334) -> (-221.695, -69.8334)
  line L1377 (-221.695, -69.8334) -> (-220.894, -69.8334)
  line L1378 (-220.894, -69.8334) -> (-220.894, -72.9326)
  line L1379 (-220.894, -72.9326) -> (-221.695, -72.9326)
  line L1380 (-257.412, -54.8831) -> (-271.413, -54.8831)
  line L1381 (-271.413, -54.8831) -> (-271.413, -50.1826)
  line L1382 (-271.413, -50.1826) -> (-272.937, -50.1826)
  line L1383 (-272.937, -50.1826) -> (-272.937, -53.4127)
  line L1384 (-272.937, -53.4127) -> (-279.688, -53.4127)
  line L1385 (-279.688, -53.4127) -> (-279.688, -50.1826)
  line L1386 (-279.688, -50.1826) -> (-280.512, -50.1826)
  line L1387 (-280.512, -50.1826) -> (-280.512, -47.3837)
  line L1388 (-280.512, -47.3837) -> (-279.688, -47.3837)
  line L1389 (-279.688, -47.3837) -> (-279.688, -41.1138)
  line L1390 (-279.688, -41.1138) -> (-277.963, -41.1138)
  line L1391 (-277.963, -41.1138) -> (-277.963, -39.9136)
  line L1392 (-277.963, -39.9136) -> (-274.662, -39.9136)
  line L1393 (-274.662, -39.9136) -> (-274.662, -41.1138)
  line L1394 (-274.662, -41.1138) -> (-272.937, -41.1138)
  line L1395 (-272.937, -41.1138) -> (-272.937, -45.5828)
  line L1396 (-272.937, -45.5828) -> (-271.413, -45.5828)
  line L1397 (-271.413, -45.5828) -> (-271.413, -40.8838)
  line L1398 (-271.413, -40.8838) -> (-257.412, -40.8838)
  line L1399 (-257.412, -40.8838) -> (-257.412, -45.5828)
  line L1400 (-257.412, -45.5828) -> (-255.888, -45.5828)
  line L1401 (-255.888, -45.5828) -> (-255.888, -41.1138)
  line L1402 (-255.888, -41.1138) -> (-254.161, -41.1138)
  line L1403 (-254.161, -41.1138) -> (-254.161, -39.9136)
  line L1404 (-254.161, -39.9136) -> (-250.862, -39.9136)
  line L1405 (-250.862, -39.9136) -> (-250.862, -41.1138)
  line L1406 (-250.862, -41.1138) -> (-249.137, -41.1138)
  line L1407 (-249.137, -41.1138) -> (-249.137, -47.3837)
  line L1408 (-249.137, -47.3837) -> (-248.313, -47.3837)
  line L1409 (-248.313, -47.3837) -> (-248.313, -50.1826)
  line L1410 (-248.313, -50.1826) -> (-249.137, -50.1826)
  line L1411 (-249.137, -50.1826) -> (-249.137, -53.4127)
  line L1412 (-249.137, -53.4127) -> (-255.888, -53.4127)
  line L1413 (-255.888, -53.4127) -> (-255.888, -50.1826)
  line L1414 (-255.888, -50.1826) -> (-257.412, -50.1826)
  line L1415 (-257.412, -50.1826) -> (-257.412, -54.8831)
  line L1416 (-312.182, -15.7827) -> (-312.182, -16.7831)
  line L1417 (-312.182, -16.7831) -> (-326.182, -16.7831)
  line L1418 (-326.182, -16.7831) -> (-326.182, -15.7827)
  line L1419 (-326.182, -15.7827) -> (-326.981, -15.7827)
  line L1420 (-326.981, -15.7827) -> (-326.981, -12.6848)
  line L1421 (-326.981, -12.6848) -> (-326.182, -12.6848)
  line L1422 (-326.182, -12.6848) -> (-326.182, -6.8833)
  line L1423 (-326.182, -6.8833) -> (-326.981, -6.8833)
  line L1424 (-326.981, -6.8833) -> (-326.981, -3.7827)
  line L1425 (-326.981, -3.7827) -> (-326.182, -3.7827)
  line L1426 (-326.182, -3.7827) -> (-326.182, -2.7836)
  line L1427 (-326.182, -2.7836) -> (-312.182, -2.7836)
  line L1428 (-312.182, -2.7836) -> (-312.182, -3.7827)
  line L1429 (-312.182, -3.7827) -> (-311.381, -3.7827)
  line L1430 (-311.381, -3.7827) -> (-311.381, -6.8833)
  line L1431 (-311.381, -6.8833) -> (-312.182, -6.8833)
  line L1432 (-312.182, -6.8833) -> (-312.182, -12.6848)
  line L1433 (-312.182, -12.6848) -> (-311.381, -12.6848)
  line L1434 (-311.381, -12.6848) -> (-311.381, -15.7827)
  line L1435 (-311.381, -15.7827) -> (-312.182, -15.7827)
  line L1436 (-312.182, -91.9826) -> (-312.182, -92.9831)
  line L1437 (-312.182, -92.9831) -> (-326.182, -92.9831)
  line L1438 (-326.182, -92.9831) -> (-326.182, -91.9826)
  line L1439 (-326.182, -91.9826) -> (-326.981, -91.9826)
  line L1440 (-326.981, -91.9826) -> (-326.981, -88.8834)
  line L1441 (-326.981, -88.8834) -> (-326.182, -88.8834)
  line L1442 (-326.182, -88.8834) -> (-326.182, -83.0834)
  line L1443 (-326.182, -83.0834) -> (-326.981, -83.0834)
  line L1444 (-326.981, -83.0834) -> (-326.981, -79.9828)
  line L1445 (-326.981, -79.9828) -> (-326.182, -79.9828)
  line L1446 (-326.182, -79.9828) -> (-326.182, -78.9838)
  line L1447 (-326.182, -78.9838) -> (-312.182, -78.9838)
  line L1448 (-312.182, -78.9838) -> (-312.182, -79.9828)
  line L1449 (-312.182, -79.9828) -> (-311.381, -79.9828)
  line L1450 (-311.381, -79.9828) -> (-311.381, -83.0834)
  line L1451 (-311.381, -83.0834) -> (-312.182, -83.0834)
  line L1452 (-312.182, -83.0834) -> (-312.182, -88.8834)
  line L1453 (-312.182, -88.8834) -> (-311.381, -88.8834)
  line L1454 (-311.381, -88.8834) -> (-311.381, -91.9826)
  line L1455 (-311.381, -91.9826) -> (-312.182, -91.9826)
  circle A0 centre (-328.707, -0.259) radius 1.1
  circle A1 centre (-247.7444, -95.6021) radius 1.1
  circle A2 centre (-171.5444, -95.6021) radius 1.1
  circle A3 centre (-192.9742, -0.259) radius 1.1
  circle A4 centre (-0.0007, -95.6021) radius 1.1
  circle A5 centre (-69.1492, -0.259) radius 1.1
  circle A6 centre (-95.3444, -95.6021) radius 1.1
  circle A7 centre (-238.2193, -58.5013) radius 1.1
  circle A8 centre (-259.6482, -0.259) radius 1.1
  circle A9 centre (-328.707, -58.5271) radius 1.1
  circle A10 centre (-287.1209, -77.5771) radius 1.1
  circle A11 centre (-162.0193, -58.4796) radius 1.1
  circle A12 centre (-128.6826, -39.4771) radius 1.1
  circle A13 centre (-0.0007, -58.4334) radius 1.1
  circle A14 centre (-0.0007, -0.259) radius 1.1
  circle A15 centre (-85.8193, -58.4579) radius 1.1
  circle A16 centre (-204.8826, -39.4771) radius 1.1
  circle A17 centre (-287.1209, -39.4771) radius 1.1
  circle A18 centre (-328.707, -95.6021) radius 1.1
  arc A19 (-328.707, 2.191) -> (-331.157, -0.259) centre (-328.707, -0.259) ccw
  line L1456 (-331.157, -0.259) -> (-331.157, -95.6021)
  arc A20 (-331.157, -95.6021) -> (-328.707, -98.0521) centre (-328.707, -95.6021) ccw
  line L1457 (-328.707, -98.0521) -> (-0.0007, -98.0521)
  arc A21 (-0.0007, -98.0521) -> (2.4493, -95.6021) centre (-0.0007, -95.6021) ccw
  line L1458 (2.4493, -95.6021) -> (2.4493, -0.259)
  arc A22 (2.4493, -0.259) -> (-0.0007, 2.191) centre (-0.0007, -0.259) ccw
  line L1459 (-0.0007, 2.191) -> (-328.707, 2.191)